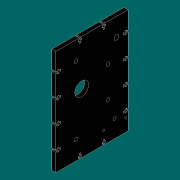
# Autodesk Inventor part: side
Saved by Autodesk Inventor 2016 (Build 200138000, 138)
## iProperties
Created: 2015-10-05
Part Number: side
Material: ABS Plastic
Document SubType Name: Modeling
Designer: Sawaiz
Density: 1.06 g/cm^3
Appearance: Smooth - Black
Author: Sawaiz
Autodesk Inventor part; units mm, degrees
ref_plane "YZ Plane" through (0, 0, 0) normal (1, 0, 0) x (0, 1, 0)
ref_plane "XZ Plane" through (0, 0, 0) normal (0, 1, 0) x (-1, 0, 0)
ref_plane "XY Plane" through (0, 0, 0) normal (0, 0, 1) x (1, 0, 0)
sketch "Sketch1" plane through (0, 0, 0) normal (1, 0, 0) x (0, 1, 0)
  line L0 (-57.5, -83.65) -> (57.5, -83.65)
  line L1 (57.5, -83.65) -> (57.5, 83.65)
  line L2 (57.5, 83.65) -> (-57.5, 83.65)
  line L3 (-57.5, 83.65) -> (-57.5, -83.65)
  line L4 (-57.5, -83.65) -> (57.5, 83.65) construction
  line L5 (57.5, -83.65) -> (-57.5, 83.65) construction
  point P0 (0, 0)
  dimension "d0" = 115
  dimension "d1" = 167.3
  constraints: 12 end point, 2 midpoint, 2 parallel, 1 horizontal, 1 perpendicular
  measures "d0" distance of L2.end L1.end
  measures "d1" distance of L1.end L0.end
extrude "Extrusion1" add sketch "Sketch1" along normal blind 6.35
sketch "Sketch2" plane through (6.35, 0, 0) normal (1, 0, 0) x (0, 0, -1)
  line L0 (83.65, -57.5) -> (83.65, 57.5) projected
  line L1 (83.65, 57.5) -> (-83.65, 57.5) projected
  line L2 (-83.65, 57.5) -> (-83.65, -57.5) projected
  line L3 (-83.65, -57.5) -> (83.65, -57.5) projected
  line L4 (-83.65, 57.5) -> (-83.65, -57.5) projected
  point P0 (0, 0)
  point P1 (-11.35, -16.35)
  dimension "d4" = 95
  dimension "d12" = 41.15
  measures "d4" distance from line of L0 point (-11.35, -16.35)
  measures "d12" distance from line of L3 point (-11.35, -16.35)
hole "Hole1" at (6.35, -16.35, 11.35) direction (-1, 0, 0) diameter 22 end through all
sketch "Sketch3" plane through (6.35, 0, 0) normal (1, 0, 0) x (0, 0, -1)
  line L0 (63.65, 18.5) -> (63.65, 53.5)
  line L1 (83.65, 57.5) -> (-83.65, 57.5) projected
  line L2 (83.65, -57.5) -> (83.65, 57.5) projected
  point P0 (0, 0)
  dimension "d13" = 35
  dimension "d14" = 4
  dimension "d15" = 20
  constraints: 2 end point, 1 vertical
  measures "d13" distance of L0.start L0.end
  measures "d14" distance from line of L1 L0.end
  measures "d15" distance from line of L2 L0.end
hole "Hole2" at (6.35, 53.5, -63.65) at (6.35, 18.5, -63.65) direction (-1, 0, 0) diameter 3 end through all
sketch "Sketch4" plane through (6.35, 0, 0) normal (1, 0, 0) x (0, 0, -1)
  circle A0 centre (63.65, 18.5) radius 1.5 projected
  point P0 (0, 0)
  point P1 (55.65, 36)
  dimension "d24" = 17.5
  dimension "d39" = 8
  measures "d24" vertical distance of point (55.65, 36) A0.centre
  measures "d39" horizontal distance of A0.centre point (55.65, 36)
hole "Hole3" at (6.35, 36, -55.65) direction (-1, 0, 0) diameter 5 end through all
sketch "Sketch6" plane through (6.35, 0, 0) normal (1, 0, 0) x (0, 0, -1)
  circle A0 centre (55.65, 36) radius 2.5 projected
  circle A1 centre (63.65, 53.5) radius 1.5 projected
  circle A2 centre (63.65, 18.5) radius 1.5 projected
  circle A3 centre (-11.35, -16.35) radius 11 projected
  line L0 (83.65, -57.5) -> (83.65, 57.5) projected
  line L1 (83.65, 57.5) -> (-83.65, 57.5) projected
  line L2 (-83.65, 57.5) -> (-83.65, -57.5) projected
  line L3 (-83.65, -57.5) -> (83.65, -57.5) projected
  line L4 (-83.65, -57.5) -> (83.65, -57.5) projected
  line L5 (-55.5, -57.5) -> (-55.5, -55.5)
  line L6 (-55.5, -55.5) -> (-56.75, -55.5)
  line L7 (-56.75, -55.5) -> (-56.75, -53)
  line L8 (-56.75, -53) -> (-55.5, -53)
  line L9 (-55.5, -53) -> (-55.5, -49.85)
  line L10 (-55.5, -49.85) -> (-52.5, -49.85)
  line L11 (-52.5, -49.85) -> (-52.5, -53)
  line L12 (-52.5, -53) -> (-51.25, -53)
  line L13 (-51.25, -53) -> (-51.25, -55.5)
  line L14 (-51.25, -55.5) -> (-52.5, -55.5)
  line L15 (-52.5, -57.5) -> (-52.5, -55.5)
  point P0 (0, 0)
  point P1 (-54, -49.85)
  dimension "d40" = 3
  dimension "d41" = 5.5
  dimension "d42" = 2.5
  dimension "d43" = 2
  dimension "d44" = 7.65
  dimension "d45" = 29.65
  constraints: 22 end point, 10 point on line, 8 perpendicular, 1 collinear, 1 midpoint
  measures "d40" distance between parallel lines of L15 L5
  measures "d41" distance between parallel lines of L7 L13
  measures "d42" distance between parallel lines of L14 L12
  measures "d43" distance between parallel lines of L3 L14
  measures "d44" distance between parallel lines of L4 L10
  measures "d45" distance from line of L2 point (-54, -49.85)
extrude "Extrusion2" cut sketch "Sketch6" against normal through all contours L3 L5 L6 L7 L8 L9 L10 L11 L12 L13 L14 L15
pattern_linear "Rectangular Pattern1" count 4 spacing 36 along (0, 0, -1) of "Extrusion2"
mirror "Mirror1" about plane through (0, 0, 0) normal (0, 1, 0) of "Extrusion2", "Rectangular Pattern1"
sketch "Sketch7" plane through (6.35, 0, 0) normal (1, 0, 0) x (0, 0, -1)
  line L0 (52.5, 55.5) -> (52.5, 57.5) projected
  line L1 (52.5, 57.5) -> (19.5, 57.5) projected
  line L2 (19.5, 57.5) -> (19.5, 55.5) projected
  line L3 (19.5, 55.5) -> (20.75, 55.5) projected
  line L4 (20.75, 55.5) -> (20.75, 53) projected
  line L5 (20.75, 53) -> (19.5, 53) projected
  line L6 (19.5, 53) -> (19.5, 49.85) projected
  line L7 (19.5, 49.85) -> (16.5, 49.85) projected
  line L8 (16.5, 49.85) -> (16.5, 53) projected
  line L9 (16.5, 53) -> (15.25, 53) projected
  line L10 (15.25, 53) -> (15.25, 55.5) projected
  line L11 (15.25, 55.5) -> (16.5, 55.5) projected
  line L12 (16.5, 55.5) -> (16.5, 57.5) projected
  line L13 (16.5, 57.5) -> (-16.5, 57.5) projected
  line L14 (-16.5, 57.5) -> (-16.5, 55.5) projected
  line L15 (-16.5, 55.5) -> (-15.25, 55.5) projected
  line L16 (-15.25, 55.5) -> (-15.25, 53) projected
  line L17 (-15.25, 53) -> (-16.5, 53) projected
  line L18 (-16.5, 53) -> (-16.5, 49.85) projected
  line L19 (-16.5, 49.85) -> (-19.5, 49.85) projected
  line L20 (-19.5, 49.85) -> (-19.5, 53) projected
  line L21 (-19.5, 53) -> (-20.75, 53) projected
  line L22 (-20.75, 53) -> (-20.75, 55.5) projected
  line L23 (-20.75, 55.5) -> (-19.5, 55.5) projected
  line L24 (-19.5, 55.5) -> (-19.5, 57.5) projected
  line L25 (-19.5, 57.5) -> (-52.5, 57.5) projected
  line L26 (-52.5, 57.5) -> (-52.5, 55.5) projected
  line L27 (-52.5, 55.5) -> (-51.25, 55.5) projected
  line L28 (-51.25, 55.5) -> (-51.25, 53) projected
  line L29 (-51.25, 53) -> (-52.5, 53) projected
  line L30 (-52.5, 53) -> (-52.5, 49.85) projected
  line L31 (-52.5, 49.85) -> (-55.5, 49.85) projected
  line L32 (-55.5, 49.85) -> (-55.5, 53) projected
  line L33 (-55.5, 53) -> (-56.75, 53) projected
  line L34 (-56.75, 53) -> (-56.75, 55.5) projected
  line L35 (-56.75, 55.5) -> (-55.5, 55.5) projected
  line L36 (-55.5, 55.5) -> (-55.5, 57.5) projected
  line L37 (-55.5, 57.5) -> (-83.65, 57.5) projected
  line L38 (-83.65, 57.5) -> (-83.65, -57.5) projected
  line L39 (-83.65, -57.5) -> (-55.5, -57.5) projected
  line L40 (-55.5, -57.5) -> (-55.5, -55.5) projected
  line L41 (-55.5, -55.5) -> (-56.75, -55.5) projected
  line L42 (-56.75, -55.5) -> (-56.75, -53) projected
  line L43 (-56.75, -53) -> (-55.5, -53) projected
  line L44 (-55.5, -53) -> (-55.5, -49.85) projected
  line L45 (-55.5, -49.85) -> (-52.5, -49.85) projected
  line L46 (-52.5, -49.85) -> (-52.5, -53) projected
  line L47 (-52.5, -53) -> (-51.25, -53) projected
  line L48 (-51.25, -53) -> (-51.25, -55.5) projected
  line L49 (-51.25, -55.5) -> (-52.5, -55.5) projected
  line L50 (-52.5, -55.5) -> (-52.5, -57.5) projected
  line L51 (-52.5, -57.5) -> (-19.5, -57.5) projected
  line L52 (-19.5, -57.5) -> (-19.5, -55.5) projected
  line L53 (-19.5, -55.5) -> (-20.75, -55.5) projected
  line L54 (-20.75, -55.5) -> (-20.75, -53) projected
  line L55 (-20.75, -53) -> (-19.5, -53) projected
  line L56 (-19.5, -53) -> (-19.5, -49.85) projected
  line L57 (-19.5, -49.85) -> (-16.5, -49.85) projected
  line L58 (-16.5, -49.85) -> (-16.5, -53) projected
  line L59 (-16.5, -53) -> (-15.25, -53) projected
  line L60 (-15.25, -53) -> (-15.25, -55.5) projected
  line L61 (-15.25, -55.5) -> (-16.5, -55.5) projected
  line L62 (-16.5, -55.5) -> (-16.5, -57.5) projected
  line L63 (-16.5, -57.5) -> (16.5, -57.5) projected
  line L64 (16.5, -57.5) -> (16.5, -55.5) projected
  line L65 (16.5, -55.5) -> (15.25, -55.5) projected
  line L66 (15.25, -55.5) -> (15.25, -53) projected
  line L67 (15.25, -53) -> (16.5, -53) projected
  line L68 (16.5, -53) -> (16.5, -49.85) projected
  line L69 (16.5, -49.85) -> (19.5, -49.85) projected
  line L70 (19.5, -49.85) -> (19.5, -53) projected
  line L71 (19.5, -53) -> (20.75, -53) projected
  line L72 (20.75, -53) -> (20.75, -55.5) projected
  line L73 (20.75, -55.5) -> (19.5, -55.5) projected
  line L74 (19.5, -55.5) -> (19.5, -57.5) projected
  line L75 (19.5, -57.5) -> (52.5, -57.5) projected
  line L76 (52.5, -57.5) -> (52.5, -55.5) projected
  line L77 (52.5, -55.5) -> (51.25, -55.5) projected
  line L78 (51.25, -55.5) -> (51.25, -53) projected
  line L79 (51.25, -53) -> (52.5, -53) projected
  line L80 (52.5, -53) -> (52.5, -49.85) projected
  line L81 (52.5, -49.85) -> (55.5, -49.85) projected
  line L82 (55.5, -49.85) -> (55.5, -53) projected
  line L83 (55.5, -53) -> (56.75, -53) projected
  line L84 (56.75, -53) -> (56.75, -55.5) projected
  line L85 (56.75, -55.5) -> (55.5, -55.5) projected
  line L86 (55.5, -55.5) -> (55.5, -57.5) projected
  line L87 (55.5, -57.5) -> (83.65, -57.5) projected
  line L88 (83.65, -57.5) -> (83.65, 57.5) projected
  line L89 (83.65, 57.5) -> (55.5, 57.5) projected
  line L90 (55.5, 57.5) -> (55.5, 55.5) projected
  line L91 (55.5, 55.5) -> (56.75, 55.5) projected
  line L92 (56.75, 55.5) -> (56.75, 53) projected
  circle A0 centre (63.65, 53.5) radius 1.5 projected
  line L93 (56.75, 53) -> (55.5, 53) projected
  line L94 (55.5, 53) -> (55.5, 49.85) projected
  line L95 (55.5, 49.85) -> (52.5, 49.85) projected
  line L96 (52.5, 49.85) -> (52.5, 53) projected
  line L97 (52.5, 53) -> (51.25, 53) projected
  line L98 (51.25, 53) -> (51.25, 55.5) projected
  line L99 (51.25, 55.5) -> (52.5, 55.5) projected
  circle A1 centre (-11.35, -16.35) radius 11 projected
  circle A2 centre (63.65, 18.5) radius 1.5 projected
  circle A3 centre (55.65, 36) radius 2.5 projected
  line L100 (-83.65, 57.5) -> (-83.65, -57.5) projected
  line L101 (-83.65, -20.6667) -> (-81.65, -20.6667)
  line L102 (-81.65, -20.6667) -> (-81.65, -21.9167)
  line L103 (-81.65, -21.9167) -> (-79.15, -21.9167)
  line L104 (-79.15, -21.9167) -> (-79.15, -20.6667)
  line L105 (-79.15, -20.6667) -> (-76, -20.6667)
  line L106 (-76, -20.6667) -> (-76, -17.6667)
  line L107 (-76, -17.6667) -> (-79.15, -17.6667)
  line L108 (-79.15, -17.6667) -> (-79.15, -16.4167)
  line L109 (-79.15, -16.4167) -> (-81.65, -16.4167)
  line L110 (-81.65, -16.4167) -> (-81.65, -17.6667)
  line L111 (-83.65, -17.6667) -> (-81.65, -17.6667)
  point P0 (0, 0)
  point P1 (-76, -19.1667)
  dimension "d51" = 5.5
  dimension "d52" = 7.65
  dimension "d53" = 2
  dimension "d54" = 3
  dimension "d55" = 38.3333
  dimension "d56" = 2.5
  constraints: 22 end point, 10 point on line, 8 perpendicular, 1 collinear, 1 midpoint
  measures "d51" distance between parallel lines of L109 L103
  measures "d52" distance between parallel lines of L100 L106
  measures "d53" distance between parallel lines of L38 L110
  measures "d54" distance between parallel lines of L105 L107
  measures "d55" distance from line of L39 point (-76, -19.167)
  measures "d56" distance between parallel lines of L104 L102
extrude "Extrusion3" cut sketch "Sketch7" against normal through all contours L111 L110 L109 L108 L107 L106 L105 L104 L103 L102 L101 L38
pattern_linear "Rectangular Pattern2" count 2 spacing 38.3333 along (0, 1, 0) of "Extrusion3"
mirror "Mirror2" about plane through (0, 0, 0) normal (0, 0, 1) of "Extrusion3", "Rectangular Pattern2"
sketch "Sketch8" plane through (6.35, 0, 0) normal (1, 0, 0) x (0, 0, -1)
  line L0 (81.65, 20.6667) -> (83.65, 20.6667) projected
  line L1 (83.65, 20.6667) -> (83.65, 57.5) projected
  line L2 (83.65, 57.5) -> (55.5, 57.5) projected
  line L3 (55.5, 57.5) -> (55.5, 55.5) projected
  line L4 (55.5, 55.5) -> (56.75, 55.5) projected
  line L5 (56.75, 55.5) -> (56.75, 53) projected
  line L6 (56.75, 53) -> (55.5, 53) projected
  line L7 (55.5, 53) -> (55.5, 49.85) projected
  line L8 (55.5, 49.85) -> (52.5, 49.85) projected
  line L9 (52.5, 49.85) -> (52.5, 53) projected
  line L10 (52.5, 53) -> (51.25, 53) projected
  line L11 (51.25, 53) -> (51.25, 55.5) projected
  line L12 (51.25, 55.5) -> (52.5, 55.5) projected
  line L13 (52.5, 55.5) -> (52.5, 57.5) projected
  line L14 (52.5, 57.5) -> (19.5, 57.5) projected
  line L15 (19.5, 57.5) -> (19.5, 55.5) projected
  line L16 (19.5, 55.5) -> (20.75, 55.5) projected
  line L17 (20.75, 55.5) -> (20.75, 53) projected
  line L18 (20.75, 53) -> (19.5, 53) projected
  line L19 (19.5, 53) -> (19.5, 49.85) projected
  line L20 (19.5, 49.85) -> (16.5, 49.85) projected
  line L21 (16.5, 49.85) -> (16.5, 53) projected
  line L22 (16.5, 53) -> (15.25, 53) projected
  line L23 (15.25, 53) -> (15.25, 55.5) projected
  line L24 (15.25, 55.5) -> (16.5, 55.5) projected
  line L25 (16.5, 55.5) -> (16.5, 57.5) projected
  line L26 (16.5, 57.5) -> (-16.5, 57.5) projected
  line L27 (-16.5, 57.5) -> (-16.5, 55.5) projected
  line L28 (-16.5, 55.5) -> (-15.25, 55.5) projected
  line L29 (-15.25, 55.5) -> (-15.25, 53) projected
  line L30 (-15.25, 53) -> (-16.5, 53) projected
  line L31 (-16.5, 53) -> (-16.5, 49.85) projected
  line L32 (-16.5, 49.85) -> (-19.5, 49.85) projected
  line L33 (-19.5, 49.85) -> (-19.5, 53) projected
  line L34 (-19.5, 53) -> (-20.75, 53) projected
  line L35 (-20.75, 53) -> (-20.75, 55.5) projected
  line L36 (-20.75, 55.5) -> (-19.5, 55.5) projected
  line L37 (-19.5, 55.5) -> (-19.5, 57.5) projected
  line L38 (-19.5, 57.5) -> (-52.5, 57.5) projected
  line L39 (-52.5, 57.5) -> (-52.5, 55.5) projected
  line L40 (-52.5, 55.5) -> (-51.25, 55.5) projected
  line L41 (-51.25, 55.5) -> (-51.25, 53) projected
  line L42 (-51.25, 53) -> (-52.5, 53) projected
  line L43 (-52.5, 53) -> (-52.5, 49.85) projected
  line L44 (-52.5, 49.85) -> (-55.5, 49.85) projected
  line L45 (-55.5, 49.85) -> (-55.5, 53) projected
  line L46 (-55.5, 53) -> (-56.75, 53) projected
  line L47 (-56.75, 53) -> (-56.75, 55.5) projected
  line L48 (-56.75, 55.5) -> (-55.5, 55.5) projected
  line L49 (-55.5, 55.5) -> (-55.5, 57.5) projected
  line L50 (-55.5, 57.5) -> (-83.65, 57.5) projected
  line L51 (-83.65, 57.5) -> (-83.65, 20.6667) projected
  line L52 (-83.65, 20.6667) -> (-81.65, 20.6667) projected
  line L53 (-81.65, 20.6667) -> (-81.65, 21.9167) projected
  line L54 (-81.65, 21.9167) -> (-79.15, 21.9167) projected
  line L55 (-79.15, 21.9167) -> (-79.15, 20.6667) projected
  line L56 (-79.15, 20.6667) -> (-76, 20.6667) projected
  line L57 (-76, 20.6667) -> (-76, 17.6667) projected
  line L58 (-76, 17.6667) -> (-79.15, 17.6667) projected
  line L59 (-79.15, 17.6667) -> (-79.15, 16.4167) projected
  line L60 (-79.15, 16.4167) -> (-81.65, 16.4167) projected
  line L61 (-81.65, 16.4167) -> (-81.65, 17.6667) projected
  line L62 (-81.65, 17.6667) -> (-83.65, 17.6667) projected
  line L63 (-83.65, 17.6667) -> (-83.65, -17.6667) projected
  line L64 (-83.65, -17.6667) -> (-81.65, -17.6667) projected
  line L65 (-81.65, -17.6667) -> (-81.65, -16.4167) projected
  line L66 (-81.65, -16.4167) -> (-79.15, -16.4167) projected
  line L67 (-79.15, -16.4167) -> (-79.15, -17.6667) projected
  line L68 (-79.15, -17.6667) -> (-76, -17.6667) projected
  line L69 (-76, -17.6667) -> (-76, -20.6667) projected
  line L70 (-76, -20.6667) -> (-79.15, -20.6667) projected
  line L71 (-79.15, -20.6667) -> (-79.15, -21.9167) projected
  line L72 (-79.15, -21.9167) -> (-81.65, -21.9167) projected
  line L73 (-81.65, -21.9167) -> (-81.65, -20.6667) projected
  line L74 (-81.65, -20.6667) -> (-83.65, -20.6667) projected
  line L75 (-83.65, -20.6667) -> (-83.65, -57.5) projected
  line L76 (-83.65, -57.5) -> (-55.5, -57.5) projected
  line L77 (-55.5, -57.5) -> (-55.5, -55.5) projected
  line L78 (-55.5, -55.5) -> (-56.75, -55.5) projected
  line L79 (-56.75, -55.5) -> (-56.75, -53) projected
  line L80 (-56.75, -53) -> (-55.5, -53) projected
  line L81 (-55.5, -53) -> (-55.5, -49.85) projected
  line L82 (-55.5, -49.85) -> (-52.5, -49.85) projected
  line L83 (-52.5, -49.85) -> (-52.5, -53) projected
  line L84 (-52.5, -53) -> (-51.25, -53) projected
  line L85 (-51.25, -53) -> (-51.25, -55.5) projected
  line L86 (-51.25, -55.5) -> (-52.5, -55.5) projected
  line L87 (-52.5, -55.5) -> (-52.5, -57.5) projected
  line L88 (-52.5, -57.5) -> (-19.5, -57.5) projected
  line L89 (-19.5, -57.5) -> (-19.5, -55.5) projected
  line L90 (-19.5, -55.5) -> (-20.75, -55.5) projected
  line L91 (-20.75, -55.5) -> (-20.75, -53) projected
  line L92 (-20.75, -53) -> (-19.5, -53) projected
  line L93 (-19.5, -53) -> (-19.5, -49.85) projected
  line L94 (-19.5, -49.85) -> (-16.5, -49.85) projected
  line L95 (-16.5, -49.85) -> (-16.5, -53) projected
  line L96 (-16.5, -53) -> (-15.25, -53) projected
  line L97 (-15.25, -53) -> (-15.25, -55.5) projected
  line L98 (-15.25, -55.5) -> (-16.5, -55.5) projected
  line L99 (-16.5, -55.5) -> (-16.5, -57.5) projected
  line L100 (-16.5, -57.5) -> (16.5, -57.5) projected
  line L101 (16.5, -57.5) -> (16.5, -55.5) projected
  line L102 (16.5, -55.5) -> (15.25, -55.5) projected
  line L103 (15.25, -55.5) -> (15.25, -53) projected
  line L104 (15.25, -53) -> (16.5, -53) projected
  line L105 (16.5, -53) -> (16.5, -49.85) projected
  line L106 (16.5, -49.85) -> (19.5, -49.85) projected
  line L107 (19.5, -49.85) -> (19.5, -53) projected
  line L108 (19.5, -53) -> (20.75, -53) projected
  line L109 (20.75, -53) -> (20.75, -55.5) projected
  line L110 (20.75, -55.5) -> (19.5, -55.5) projected
  line L111 (19.5, -55.5) -> (19.5, -57.5) projected
  line L112 (19.5, -57.5) -> (52.5, -57.5) projected
  line L113 (52.5, -57.5) -> (52.5, -55.5) projected
  line L114 (52.5, -55.5) -> (51.25, -55.5) projected
  line L115 (51.25, -55.5) -> (51.25, -53) projected
  line L116 (51.25, -53) -> (52.5, -53) projected
  line L117 (52.5, -53) -> (52.5, -49.85) projected
  line L118 (52.5, -49.85) -> (55.5, -49.85) projected
  line L119 (55.5, -49.85) -> (55.5, -53) projected
  line L120 (55.5, -53) -> (56.75, -53) projected
  line L121 (56.75, -53) -> (56.75, -55.5) projected
  line L122 (56.75, -55.5) -> (55.5, -55.5) projected
  line L123 (55.5, -55.5) -> (55.5, -57.5) projected
  line L124 (55.5, -57.5) -> (83.65, -57.5) projected
  line L125 (83.65, -57.5) -> (83.65, -20.6667) projected
  line L126 (83.65, -20.6667) -> (81.65, -20.6667) projected
  line L127 (81.65, -20.6667) -> (81.65, -21.9167) projected
  line L128 (81.65, -21.9167) -> (79.15, -21.9167) projected
  line L129 (79.15, -21.9167) -> (79.15, -20.6667) projected
  line L130 (79.15, -20.6667) -> (76, -20.6667) projected
  line L131 (76, -20.6667) -> (76, -17.6667) projected
  line L132 (76, -17.6667) -> (79.15, -17.6667) projected
  line L133 (79.15, -17.6667) -> (79.15, -16.4167) projected
  line L134 (79.15, -16.4167) -> (81.65, -16.4167) projected
  line L135 (81.65, -16.4167) -> (81.65, -17.6667) projected
  line L136 (81.65, -17.6667) -> (83.65, -17.6667) projected
  line L137 (83.65, -17.6667) -> (83.65, 17.6667) projected
  line L138 (83.65, 17.6667) -> (81.65, 17.6667) projected
  line L139 (81.65, 17.6667) -> (81.65, 16.4167) projected
  line L140 (81.65, 16.4167) -> (79.15, 16.4167) projected
  line L141 (79.15, 16.4167) -> (79.15, 17.6667) projected
  line L142 (79.15, 17.6667) -> (76, 17.6667) projected
  line L143 (76, 17.6667) -> (76, 20.6667) projected
  line L144 (76, 20.6667) -> (79.15, 20.6667) projected
  line L145 (79.15, 20.6667) -> (79.15, 21.9167) projected
  line L146 (79.15, 21.9167) -> (81.65, 21.9167) projected
  line L147 (81.65, 21.9167) -> (81.65, 20.6667) projected
  circle A0 centre (-11.35, -16.35) radius 11 projected
  circle A1 centre (63.65, 18.5) radius 1.5 projected
  circle A2 centre (63.65, 53.5) radius 1.5 projected
  circle A3 centre (55.65, 36) radius 2.5 projected
  circle A4 centre (-54.7671, 39.0294) radius 4 projected
  point P0 (0, 0)
  constraints: 1 coincident
hole "Hole5" at (6.35, 39.0294, 54.7671) direction (-1, 0, 0) diameter 8 end through all
sketch "Sketch9" plane through (6.35, 0, 0) normal (1, 0, 0) x (0, 0, -1)
  circle A0 centre (-54.7671, 39.0294) radius 4 projected
  line L0 (81.65, 20.6667) -> (83.65, 20.6667) projected
  line L1 (83.65, 20.6667) -> (83.65, 57.5) projected
  line L2 (83.65, 57.5) -> (55.5, 57.5) projected
  line L3 (55.5, 57.5) -> (55.5, 55.5) projected
  line L4 (55.5, 55.5) -> (56.75, 55.5) projected
  line L5 (56.75, 55.5) -> (56.75, 53) projected
  line L6 (56.75, 53) -> (55.5, 53) projected
  line L7 (55.5, 53) -> (55.5, 49.85) projected
  line L8 (55.5, 49.85) -> (52.5, 49.85) projected
  line L9 (52.5, 49.85) -> (52.5, 53) projected
  line L10 (52.5, 53) -> (51.25, 53) projected
  line L11 (51.25, 53) -> (51.25, 55.5) projected
  line L12 (51.25, 55.5) -> (52.5, 55.5) projected
  line L13 (52.5, 55.5) -> (52.5, 57.5) projected
  line L14 (52.5, 57.5) -> (19.5, 57.5) projected
  line L15 (19.5, 57.5) -> (19.5, 55.5) projected
  line L16 (19.5, 55.5) -> (20.75, 55.5) projected
  line L17 (20.75, 55.5) -> (20.75, 53) projected
  line L18 (20.75, 53) -> (19.5, 53) projected
  line L19 (19.5, 53) -> (19.5, 49.85) projected
  line L20 (19.5, 49.85) -> (16.5, 49.85) projected
  line L21 (16.5, 49.85) -> (16.5, 53) projected
  line L22 (16.5, 53) -> (15.25, 53) projected
  line L23 (15.25, 53) -> (15.25, 55.5) projected
  line L24 (15.25, 55.5) -> (16.5, 55.5) projected
  line L25 (16.5, 55.5) -> (16.5, 57.5) projected
  line L26 (16.5, 57.5) -> (-16.5, 57.5) projected
  line L27 (-16.5, 57.5) -> (-16.5, 55.5) projected
  line L28 (-16.5, 55.5) -> (-15.25, 55.5) projected
  line L29 (-15.25, 55.5) -> (-15.25, 53) projected
  line L30 (-15.25, 53) -> (-16.5, 53) projected
  line L31 (-16.5, 53) -> (-16.5, 49.85) projected
  line L32 (-16.5, 49.85) -> (-19.5, 49.85) projected
  line L33 (-19.5, 49.85) -> (-19.5, 53) projected
  line L34 (-19.5, 53) -> (-20.75, 53) projected
  line L35 (-20.75, 53) -> (-20.75, 55.5) projected
  line L36 (-20.75, 55.5) -> (-19.5, 55.5) projected
  line L37 (-19.5, 55.5) -> (-19.5, 57.5) projected
  line L38 (-19.5, 57.5) -> (-52.5, 57.5) projected
  line L39 (-52.5, 57.5) -> (-52.5, 55.5) projected
  line L40 (-52.5, 55.5) -> (-51.25, 55.5) projected
  line L41 (-51.25, 55.5) -> (-51.25, 53) projected
  line L42 (-51.25, 53) -> (-52.5, 53) projected
  line L43 (-52.5, 53) -> (-52.5, 49.85) projected
  line L44 (-52.5, 49.85) -> (-55.5, 49.85) projected
  line L45 (-55.5, 49.85) -> (-55.5, 53) projected
  line L46 (-55.5, 53) -> (-56.75, 53) projected
  line L47 (-56.75, 53) -> (-56.75, 55.5) projected
  line L48 (-56.75, 55.5) -> (-55.5, 55.5) projected
  line L49 (-55.5, 55.5) -> (-55.5, 57.5) projected
  line L50 (-55.5, 57.5) -> (-83.65, 57.5) projected
  line L51 (-83.65, 57.5) -> (-83.65, 20.6667) projected
  line L52 (-83.65, 20.6667) -> (-81.65, 20.6667) projected
  line L53 (-81.65, 20.6667) -> (-81.65, 21.9167) projected
  line L54 (-81.65, 21.9167) -> (-79.15, 21.9167) projected
  line L55 (-79.15, 21.9167) -> (-79.15, 20.6667) projected
  line L56 (-79.15, 20.6667) -> (-76, 20.6667) projected
  line L57 (-76, 20.6667) -> (-76, 17.6667) projected
  line L58 (-76, 17.6667) -> (-79.15, 17.6667) projected
  line L59 (-79.15, 17.6667) -> (-79.15, 16.4167) projected
  line L60 (-79.15, 16.4167) -> (-81.65, 16.4167) projected
  line L61 (-81.65, 16.4167) -> (-81.65, 17.6667) projected
  line L62 (-81.65, 17.6667) -> (-83.65, 17.6667) projected
  line L63 (-83.65, 17.6667) -> (-83.65, -17.6667) projected
  line L64 (-83.65, -17.6667) -> (-81.65, -17.6667) projected
  line L65 (-81.65, -17.6667) -> (-81.65, -16.4167) projected
  line L66 (-81.65, -16.4167) -> (-79.15, -16.4167) projected
  line L67 (-79.15, -16.4167) -> (-79.15, -17.6667) projected
  line L68 (-79.15, -17.6667) -> (-76, -17.6667) projected
  line L69 (-76, -17.6667) -> (-76, -20.6667) projected
  line L70 (-76, -20.6667) -> (-79.15, -20.6667) projected
  line L71 (-79.15, -20.6667) -> (-79.15, -21.9167) projected
  line L72 (-79.15, -21.9167) -> (-81.65, -21.9167) projected
  line L73 (-81.65, -21.9167) -> (-81.65, -20.6667) projected
  line L74 (-81.65, -20.6667) -> (-83.65, -20.6667) projected
  line L75 (-83.65, -20.6667) -> (-83.65, -57.5) projected
  line L76 (-83.65, -57.5) -> (-55.5, -57.5) projected
  line L77 (-55.5, -57.5) -> (-55.5, -55.5) projected
  line L78 (-55.5, -55.5) -> (-56.75, -55.5) projected
  line L79 (-56.75, -55.5) -> (-56.75, -53) projected
  line L80 (-56.75, -53) -> (-55.5, -53) projected
  line L81 (-55.5, -53) -> (-55.5, -49.85) projected
  line L82 (-55.5, -49.85) -> (-52.5, -49.85) projected
  line L83 (-52.5, -49.85) -> (-52.5, -53) projected
  line L84 (-52.5, -53) -> (-51.25, -53) projected
  line L85 (-51.25, -53) -> (-51.25, -55.5) projected
  line L86 (-51.25, -55.5) -> (-52.5, -55.5) projected
  line L87 (-52.5, -55.5) -> (-52.5, -57.5) projected
  line L88 (-52.5, -57.5) -> (-19.5, -57.5) projected
  line L89 (-19.5, -57.5) -> (-19.5, -55.5) projected
  line L90 (-19.5, -55.5) -> (-20.75, -55.5) projected
  line L91 (-20.75, -55.5) -> (-20.75, -53) projected
  line L92 (-20.75, -53) -> (-19.5, -53) projected
  line L93 (-19.5, -53) -> (-19.5, -49.85) projected
  line L94 (-19.5, -49.85) -> (-16.5, -49.85) projected
  line L95 (-16.5, -49.85) -> (-16.5, -53) projected
  line L96 (-16.5, -53) -> (-15.25, -53) projected
  line L97 (-15.25, -53) -> (-15.25, -55.5) projected
  line L98 (-15.25, -55.5) -> (-16.5, -55.5) projected
  line L99 (-16.5, -55.5) -> (-16.5, -57.5) projected
  line L100 (-16.5, -57.5) -> (16.5, -57.5) projected
  line L101 (16.5, -57.5) -> (16.5, -55.5) projected
  line L102 (16.5, -55.5) -> (15.25, -55.5) projected
  line L103 (15.25, -55.5) -> (15.25, -53) projected
  line L104 (15.25, -53) -> (16.5, -53) projected
  line L105 (16.5, -53) -> (16.5, -49.85) projected
  line L106 (16.5, -49.85) -> (19.5, -49.85) projected
  line L107 (19.5, -49.85) -> (19.5, -53) projected
  line L108 (19.5, -53) -> (20.75, -53) projected
  line L109 (20.75, -53) -> (20.75, -55.5) projected
  line L110 (20.75, -55.5) -> (19.5, -55.5) projected
  line L111 (19.5, -55.5) -> (19.5, -57.5) projected
  line L112 (19.5, -57.5) -> (52.5, -57.5) projected
  line L113 (52.5, -57.5) -> (52.5, -55.5) projected
  line L114 (52.5, -55.5) -> (51.25, -55.5) projected
  line L115 (51.25, -55.5) -> (51.25, -53) projected
  line L116 (51.25, -53) -> (52.5, -53) projected
  line L117 (52.5, -53) -> (52.5, -49.85) projected
  line L118 (52.5, -49.85) -> (55.5, -49.85) projected
  line L119 (55.5, -49.85) -> (55.5, -53) projected
  line L120 (55.5, -53) -> (56.75, -53) projected
  line L121 (56.75, -53) -> (56.75, -55.5) projected
  line L122 (56.75, -55.5) -> (55.5, -55.5) projected
  line L123 (55.5, -55.5) -> (55.5, -57.5) projected
  line L124 (55.5, -57.5) -> (83.65, -57.5) projected
  line L125 (83.65, -57.5) -> (83.65, -20.6667) projected
  line L126 (83.65, -20.6667) -> (81.65, -20.6667) projected
  line L127 (81.65, -20.6667) -> (81.65, -21.9167) projected
  line L128 (81.65, -21.9167) -> (79.15, -21.9167) projected
  line L129 (79.15, -21.9167) -> (79.15, -20.6667) projected
  line L130 (79.15, -20.6667) -> (76, -20.6667) projected
  line L131 (76, -20.6667) -> (76, -17.6667) projected
  line L132 (76, -17.6667) -> (79.15, -17.6667) projected
  line L133 (79.15, -17.6667) -> (79.15, -16.4167) projected
  line L134 (79.15, -16.4167) -> (81.65, -16.4167) projected
  line L135 (81.65, -16.4167) -> (81.65, -17.6667) projected
  line L136 (81.65, -17.6667) -> (83.65, -17.6667) projected
  line L137 (83.65, -17.6667) -> (83.65, 17.6667) projected
  line L138 (83.65, 17.6667) -> (81.65, 17.6667) projected
  line L139 (81.65, 17.6667) -> (81.65, 16.4167) projected
  line L140 (81.65, 16.4167) -> (79.15, 16.4167) projected
  line L141 (79.15, 16.4167) -> (79.15, 17.6667) projected
  line L142 (79.15, 17.6667) -> (76, 17.6667) projected
  line L143 (76, 17.6667) -> (76, 20.6667) projected
  line L144 (76, 20.6667) -> (79.15, 20.6667) projected
  line L145 (79.15, 20.6667) -> (79.15, 21.9167) projected
  line L146 (79.15, 21.9167) -> (81.65, 21.9167) projected
  line L147 (81.65, 21.9167) -> (81.65, 20.6667) projected
  circle A1 centre (-11.35, -16.35) radius 11 projected
  circle A2 centre (63.65, 18.5) radius 1.5 projected
  circle A3 centre (63.65, 53.5) radius 1.5 projected
  circle A4 centre (55.65, 36) radius 2.5 projected
  line L148 (54, -25.5167) -> (-54, -25.5167)
  line L149 (-54, -25.5167) -> (-24.5359, 25.5167)
  line L150 (-24.5359, 25.5167) -> (24.5359, 25.5167)
  line L151 (24.5359, 25.5167) -> (54, -25.5167)
  point P0 (0, 0)
  dimension "d71" = 29.65
  dimension "d72" = 29.65
  dimension "d73" = 31.9833
  dimension "d74" = 60
  dimension "d75" = 60
  dimension "d76" = 31.9833
  constraints: 8 end point, 2 horizontal
  measures "d71" distance from line of L75 L148.end
  measures "d72" distance from line of L125 L148.start
  measures "d73" distance between parallel lines of L112 L148
  measures "d74" angle of L148 L149
  measures "d75" angle of L148 L151
  measures "d76" distance between parallel lines of L26 L150
hole "Hole6" at (6.35, -25.5167, 54) at (6.35, 25.5167, 24.5359) at (6.35, 25.5167, -24.5359) at (6.35, -25.5167, -54) direction (-1, 0, 0) diameter 6 end through all
equation "\"d0\" = depth"
equation "\"d1\" = height - 2 * materialThickness"
equation "\"d2\" = materialThickness"
equation "\"d4\" = axleHeight"
equation "\"d12\" = 0.5 * spoolDiameter - materialThickness"
equation "\"d5\" = bearingOd"
equation "\"d41\" = nutTrapwidth"
equation "\"d42\" = nutTrapDepth"
equation "\"d43\" = nutTrapClearence"
equation "\"d45\" = 0.2 * height - materialThickness"
equation "\"d50\" = 0.2 * height"
equation "\"d51\" = nutTrapwidth"
equation "\"d53\" = nutTrapClearence"
equation "\"d55\" = 0.333333 * depth"
equation "\"d56\" = nutTrapDepth"
equation "\"d61\" = 0.333333 * depth"
equation "\"d62\" = centeralShaftDiameter"
equation "\"d71\" = 0.2 * height - materialThickness"
equation "\"d72\" = 0.2 * height - materialThickness"
equation "\"d73\" = 0.333333 * depth - materialThickness"
equation "\"d76\" = 0.333333 * depth - materialThickness"
equation "\"d77\" = magnetDiameter"
equation "\"depth\" = 115"
equation "\"materialThickness\" = 6.35"
equation "\"laserKerf\" = 0.1"
equation "\"cardPinDiameter\" = 3"
equation "\"spoolDiameter\" = 95"
equation "\"cardHeight\" = 53.98"
equation "\"cardSelected\" = 1"
equation "\"cardFillet\" = 2.88"
equation "\"centeralShaftDiameter\" = 8"
equation "\"cardThickness\" = 0.76"
equation "\"cardWidth\" = 85.6"
equation "\"cardClearence\" = 0.5"
equation "\"bearingWidth\" = 8"
equation "\"bearingOd\" = 22"
equation "\"axleHeight\" = 95"
equation "\"nutTrapDepth\" = 2.5"
equation "\"nutTrapClearence\" = 2"
equation "\"nutTrapwidth\" = 5.5"
equation "\"magnetDiameter\" = 6"
equation "\"magnetProtusion\" = 0.25"
equation "\"height\" = 180"
body "Solid1"
